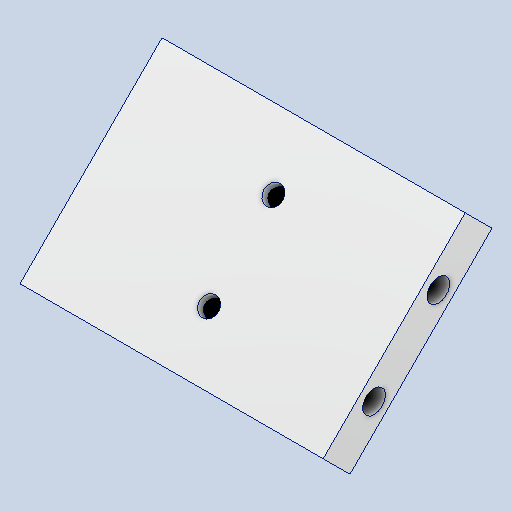
# Autodesk Inventor part: belt_liner_v1_Plate_7
Saved by Autodesk Inventor 2025.2 (Build 292293000, 293)
## iProperties
Created: 2024-12-08
Part Number: belt_liner_v1_Plate_7
Material: アルミニウム 6061
Document SubType Name: Modeling
Designer: haruy
Density: 2.7 g/cm^3
Appearance: アルミニウム - フラット
Author: haruy
Autodesk Inventor part; units mm, degrees
ref_plane "YZ Plane" through (0, 0, 0) normal (1, 0, 0) x (0, 1, 0)
ref_plane "XZ Plane" through (0, 0, 0) normal (0, 1, 0) x (-1, 0, 0)
ref_plane "XY Plane" through (0, 0, 0) normal (0, 0, 1) x (1, 0, 0)
derived "belt_liner_v1_Sketch_Base.ipt"
ref_plane "作業平面3" through (0, 300, 0) normal (0, 1, 0) x (-1, 0, 0)
sketch "スケッチ1" plane through (300, 0, 0) normal (1, 0, 0) x (0, 1, 0)
  circle A0 centre (0, 0) radius 23.875 projected
  circle A1 centre (323.2892, -323.2892) radius 23.875 projected
  line L0 (0, 0) -> (0, -985.832) projected
  line L1 (14.1421, 50.3106) -> (24.7487, 60.9172) projected
  line L2 (24.7487, 60.9172) -> (406.5864, -320.9204) projected
  line L3 (406.5864, -320.9204) -> (395.9798, -331.527) projected
  line L4 (395.9798, -331.527) -> (14.1421, 50.3106) projected
  line L5 (0, 0) -> (323.2892, -323.2892) projected
  line L6 (-50.3106, -14.1421) -> (-60.9172, -24.7487) projected
  line L7 (-60.9172, -24.7487) -> (289.1006, -374.7666) projected
  line L8 (289.1006, -374.7666) -> (299.7072, -364.16) projected
  line L9 (299.7072, -364.16) -> (-50.3106, -14.1421) projected
  line L10 (22.5524, 63.1136) -> (22.5524, 63.1136) projected
  line L11 (14.1421, 50.3106) -> (71.3109, -6.8581) projected
  line L12 (71.3109, -6.8581) -> (67.7754, -10.3937) projected
  line L13 (67.7754, -10.3937) -> (10.6066, 46.7751) projected
  line L14 (10.6066, 46.7751) -> (14.1421, 50.3106) projected
  line L15 (395.9798, -331.527) -> (376.5344, -312.0816) projected
  line L16 (376.5344, -312.0816) -> (372.9988, -315.6171) construction
  line L17 (372.9988, -315.6171) -> (392.4443, -335.0625) construction
  line L18 (392.4443, -335.0625) -> (395.9798, -331.527) projected
  line L19 (0, -985.832) -> (0, 0) projected
  circle A2 centre (0, 0) radius 12.5 projected
  circle A3 centre (21.2132, -21.2132) radius 23.5 construction
  circle A4 centre (0, 0) radius 15 projected
  circle A5 centre (21.2132, -21.2132) radius 15 projected
  line L20 (0, 0) -> (0, 0) projected
  circle A6 centre (-21.2132, 21.2132) radius 15 construction
  circle A7 centre (-21.2132, 21.2132) radius 12.25 construction
  circle A8 centre (0, 0) radius 25.575 construction
  line L21 (0, 0) -> (0, 0) projected
  line L22 (0, 0) -> (0, 0) projected
  circle A9 centre (52.7132, -21.2132) radius 1.5 projected
  circle A10 centre (21.2132, -21.2132) radius 31.5 construction
  line L23 (21.2132, -21.2132) -> (49.9041, 7.4777) projected
  circle A11 centre (21.2132, 10.2868) radius 1.5 projected
  circle A12 centre (-10.2868, -21.2132) radius 1.5 projected
  circle A13 centre (21.2132, -52.7132) radius 1.5 projected
  circle A14 centre (21.2132, -52.7132) radius 3 construction
  circle A15 centre (52.7132, -21.2132) radius 3 construction
  circle A16 centre (21.2132, -52.7132) radius 3 construction
  circle A17 centre (-10.2868, -21.2132) radius 3 construction
  circle A18 centre (21.2132, 10.2868) radius 3 construction
  line L24 (23.3345, 12.4081) -> (54.8345, -19.0919) construction
  line L25 (54.8345, -23.3345) -> (23.3345, -54.8345) construction
  line L26 (19.0919, -54.8345) -> (-12.4081, -23.3345) construction
  line L27 (-50.3106, -14.1421) -> (-46.7751, -10.6066) projected
  line L28 (-46.7751, -10.6066) -> (10.3937, -67.7754) projected
  line L29 (10.3937, -67.7754) -> (6.8581, -71.3109) projected
  line L30 (6.8581, -71.3109) -> (-50.3106, -14.1421) projected
  line L31 (-15.7223, 32.1636) -> (22.5579, 12.9685) construction
  line L32 (-32.1636, 15.7223) -> (-12.9685, -22.5579) construction
  line L33 (84.8528, 0.8132) -> (406.5864, -320.9204) projected
  line L34 (406.5864, -320.9204) -> (410.4755, -317.0313) projected
  line L35 (410.4755, -317.0313) -> (88.7419, 4.7023) projected
  line L36 (88.7419, 4.7023) -> (84.8528, 0.8132) projected
  circle A19 centre (323.2892, -323.2892) radius 5 projected
  line L37 (299.7072, -364.16) -> (280.9689, -345.4217) projected
  line L38 (280.9689, -345.4217) -> (284.5044, -341.8861) projected
  line L39 (284.5044, -341.8861) -> (303.2427, -360.6245) projected
  line L40 (303.2427, -360.6245) -> (299.7072, -364.16) projected
  circle A20 centre (319.7537, -319.7537) radius 5.1 projected
  line L41 (323.2892, -323.2892) -> (417.2615, -417.2615) projected
  circle A21 centre (337.4314, -337.4314) radius 5.1 projected
  line L42 (323.3599, -316.1474) -> (341.0376, -333.8251) projected
  line L43 (316.1474, -323.3599) -> (333.8251, -341.0376) projected
  circle A22 centre (323.2892, -323.2892) radius 22.175 projected
  circle A23 centre (323.2892, -323.2892) radius 33.875 projected
  line L44 (374.5443, -310.0916) -> (356.8667, -327.7692) projected
  line L45 (356.8667, -327.7692) -> (363.9377, -334.8403) projected
  line L46 (363.9377, -334.8403) -> (381.6154, -317.1626) projected
  line L47 (381.6154, -317.1626) -> (374.5443, -310.0916) projected
  circle A24 centre (319.7537, -319.7537) radius 10.1 projected
  circle A25 centre (337.4314, -337.4314) radius 10.1 projected
  line L48 (326.8955, -312.6119) -> (344.5731, -330.2896) projected
  line L49 (312.6119, -326.8955) -> (330.2896, -344.5731) projected
  line L50 (326.8955, -312.6119) -> (318.3599, -304.0764) projected
  line L51 (312.6119, -312.6119) -> (319.7537, -305.4701) projected
  line L52 (319.7537, -305.4701) -> (376.5344, -312.0816) construction
  line L53 (392.4443, -335.0625) -> (303.2427, -360.6245) construction
  line L54 (344.5731, -330.2896) -> (351.3689, -337.0853) projected
  line L55 (351.3689, -337.0853) -> (351.6442, -337.3606) projected
  line L56 (71.3109, -6.8581) -> (67.7754, -10.3937) projected
  line L57 (67.7754, -10.3937) -> (90.8632, -33.4815) projected
  line L58 (90.8632, -33.4815) -> (94.3988, -29.946) projected
  line L59 (94.3988, -29.946) -> (71.3109, -6.8581) projected
  line L60 (244.0828, -334.7487) -> (-45.9172, -334.7487) projected
  line L61 (-45.9172, -334.7487) -> (-45.9172, -349.7487) projected
  line L62 (-45.9172, -349.7487) -> (244.0828, -349.7487) projected
  line L63 (244.0828, -349.7487) -> (244.0828, -334.7487) projected
  line L64 (-60.9172, -24.7487) -> (-60.9172, -604.2835) projected
  line L65 (-45.9172, -334.7487) -> (-60.9172, -334.7487) projected
  line L66 (-60.9172, -334.7487) -> (-60.9172, -349.7487) projected
  line L67 (-60.9172, -349.7487) -> (-45.9172, -349.7487) projected
  line L68 (-45.9172, -349.7487) -> (-45.9172, -334.7487) projected
  line L69 (-60.9172, -334.7487) -> (-45.9172, -334.7487) projected
  line L70 (-45.9172, -334.7487) -> (-45.9172, -44.7487) projected
  line L71 (-45.9172, -44.7487) -> (-60.9172, -44.7487) projected
  line L72 (-60.9172, -44.7487) -> (-60.9172, -334.7487) projected
  line L73 (330.2896, -344.5731) -> (344.5731, -330.2896) projected
  line L74 (344.5731, -330.2896) -> (351.6442, -337.3606) projected
  line L75 (351.6442, -337.3606) -> (337.3606, -351.6442) projected
  line L76 (337.3606, -351.6442) -> (330.2896, -344.5731) projected
  line L77 (406.5864, -320.9204) -> (395.9798, -331.527) projected
  line L78 (395.9798, -331.527) -> (410.1219, -345.6691) projected
  line L79 (410.1219, -345.6691) -> (420.7285, -335.0625) projected
  line L80 (420.7285, -335.0625) -> (406.5864, -320.9204) projected
  line L81 (-12.1904, 2.7649) -> (-50.3106, -35.3553) projected
  line L82 (-12.1904, 2.7649) -> (35.3553, 50.3106) projected
  line L83 (6.8581, -71.3109) -> (-3.7485, -81.9175) projected
  line L84 (-22.0264, -35.3553) -> (-36.1685, -49.4975) construction
  line L85 (-0.8132, -56.5685) -> (-14.9553, -70.7107) projected
  circle A26 centre (-30.8652, -30.052) radius 1.5 construction
  circle A27 centre (-13.1875, -47.7297) radius 1.5 construction
  circle A28 centre (2.7224, -63.6396) radius 1.5 construction
  line L86 (49.4975, 36.1685) -> (35.3553, 22.0264) projected
  line L87 (70.7107, 14.9553) -> (56.5685, 0.8132) projected
  circle A29 centre (40.6586, 20.2586) radius 1.5 projected
  circle A30 centre (58.3363, 2.5809) radius 1.5 projected
  circle A31 centre (63.6396, -2.7224) radius 1.5 construction
  line L88 (289.4542, -346.8359) -> (285.9186, -350.3714) projected
  line L89 (297.9394, -355.3212) -> (294.4039, -358.8567) projected
  circle A32 centre (287.6864, -348.6036) radius 1.5 projected
  circle A33 centre (296.1717, -357.0889) radius 1.5 projected
  line L90 (381.4841, -317.0313) -> (377.9486, -320.5669) construction
  line L91 (389.9694, -325.5166) -> (386.4339, -329.0521) construction
  circle A34 centre (379.7163, -318.7991) radius 1.5 construction
  circle A35 centre (388.2016, -327.2844) radius 1.5 construction
  line L92 (284.5044, -341.8861) -> (312.4678, -312.7589) projected
  line L93 (312.6119, -326.8955) -> (305.4745, -320.0433) projected
  circle A36 centre (333.8958, -323.1478) radius 1.25 projected
  circle A37 centre (323.1478, -333.8958) radius 1.25 projected
  line L94 (-45.9172, -64.7487) -> (-60.9172, -64.7487) projected
  line L95 (-10.3106, -54.1421) -> (-20.9172, -64.7487) projected
  line L96 (-20.9172, -64.7487) -> (-45.9172, -64.7487) projected
  line L97 (224.0828, -334.7487) -> (224.0828, -349.7487) projected
  line L98 (244.0828, -349.7487) -> (264.0828, -349.7487) projected
  line L99 (264.0828, -349.7487) -> (274.6894, -339.1421) projected
  line L100 (244.0828, -334.7487) -> (249.0828, -334.7487) projected
  line L101 (249.0828, -334.7487) -> (259.6894, -324.1421) projected
  line L102 (-45.9172, -44.7487) -> (-40.9172, -44.7487) projected
  line L103 (-40.9172, -44.7487) -> (-30.3106, -34.1421) projected
  line L104 (-45.9172, -329.7487) -> (-60.9172, -329.7487) projected
  line L105 (-25.9172, -334.7487) -> (-25.9172, -349.7487) projected
  line L106 (-24.8548, -32.5269) -> (-38.9969, -46.669) projected
  circle A38 centre (0, 0) radius 45 projected
  circle A39 centre (56.9618, -18.8508) radius 22 projected
  circle A40 centre (56.9618, -18.8508) radius 15 projected
  circle A41 centre (79.5495, -33.4815) radius 3 projected
  circle A42 centre (39.0845, -39.0845) radius 3 projected
  circle A43 centre (39.0845, -39.0845) radius 4 projected
  circle A44 centre (18.8508, -56.9618) radius 22 projected
  circle A45 centre (18.8508, -56.9618) radius 15 projected
  circle A46 centre (33.4815, -79.5495) radius 3 projected
  circle A47 centre (39.0845, -39.0845) radius 3 projected
  line L107 (10.3937, -67.7754) -> (6.8581, -71.3109) projected
  line L108 (6.8581, -71.3109) -> (29.946, -94.3988) projected
  line L109 (29.946, -94.3988) -> (33.4815, -90.8632) projected
  line L110 (33.4815, -90.8632) -> (10.3937, -67.7754) projected
  line L111 (90.8632, -33.4815) -> (33.4815, -90.8632) projected
  circle A48 centre (76.014, -15.0967) radius 1.5 projected
  circle A49 centre (-20.2586, -40.6586) radius 1.5 projected
  circle A50 centre (-2.5809, -58.3363) radius 1.5 projected
  circle A51 centre (15.0967, -76.014) radius 1.5 projected
  circle A52 centre (323.2892, -323.2892) radius 6 projected
  circle A53 centre (0, 0) radius 25.575 construction
  circle A54 centre (0, 0) radius 25.525 projected
  circle A55 centre (323.2892, -323.2892) radius 25.525 projected
  line L112 (341.3381, -305.2403) -> (18.0489, 18.0489) projected
  circle A56 centre (309.7835, -309.7835) radius 4 projected
  circle A57 centre (309.7835, -309.7835) radius 1.25 projected
  circle A58 centre (323.2892, -323.2892) radius 18.525 projected
  circle A59 centre (332.5523, -314.1675) radius 4 projected
  line L113 (316.2182, -330.5017) -> (323.3599, -323.3599) projected
  circle A60 centre (332.5523, -314.1675) radius 1.25 projected
  line L114 (319.7537, -305.4701) -> (324.6327, -300.5911) projected
  line L115 (324.6327, -300.5911) -> (356.5232, -332.4816) projected
  line L116 (351.6442, -337.3606) -> (356.5232, -332.4816) projected
  line L117 (324.6327, -300.5911) -> (308.513, -305.9906) projected
  line L118 (300.5911, -324.6327) -> (332.4816, -356.5232) projected
  line L119 (300.5911, -324.6327) -> (305.9906, -308.513) projected
  line L120 (337.3606, -351.6442) -> (332.4816, -356.5232) projected
  circle A61 centre (314.1675, -332.5523) radius 4 projected
  circle A62 centre (314.1675, -332.5523) radius 1.25 projected
  line L121 (88.7419, 4.7023) -> (131.1683, -37.7241) projected
  line L122 (131.1683, -37.7241) -> (134.3503, -34.5422) projected
  line L123 (134.3503, -34.5422) -> (91.9239, 7.8842) projected
  line L124 (91.9239, 7.8842) -> (88.7419, 4.7023) projected
  circle A63 centre (258.094, 18.4908) radius 120 projected
  line L125 (134.3503, -34.5422) -> (77.7817, 22.0264) projected
  line L126 (77.7817, 22.0264) -> (81.3173, 25.5619) projected
  line L127 (81.3173, 25.5619) -> (137.8858, -31.0066) projected
  line L128 (137.8858, -31.0066) -> (134.3503, -34.5422) projected
  line L129 (76.7211, -47.6236) -> (112.0764, -12.2683) construction
  line L130 (112.0764, -12.2683) -> (119.1475, -19.3394) projected
  line L131 (119.1475, -19.3394) -> (83.7922, -54.6947) construction
  line L132 (83.7922, -54.6947) -> (76.7211, -47.6236) construction
  line L133 (258.094, 18.4908) -> (258.094, 138.4908) projected
  line L134 (258.094, 18.4908) -> (173.2412, 103.3437) projected
  line L135 (258.094, 18.4908) -> (138.094, 18.4908) projected
  line L136 (77.7817, 22.0264) -> (94.3988, -29.946) construction
  circle A64 centre (258.094, 18.4908) radius 130 projected
  line L137 (81.3173, 25.5619) -> (267.9719, 212.2165) projected
  line L138 (258.094, 138.4908) -> (138.094, 18.4908) projected
  line L139 (258.094, 138.4908) -> (258.094, 148.4908) projected
  line L140 (258.094, 18.4908) -> (166.1701, -73.433) projected
  line L141 (173.2412, -66.362) -> (166.1701, -73.433) projected
  line L142 (166.1701, -73.433) -> (180.3122, -87.5752) projected
  line L143 (180.3122, -87.5752) -> (187.3833, -80.5041) projected
  line L144 (187.3833, -80.5041) -> (173.2412, -66.362) projected
  line L145 (180.3122, -87.5752) -> (101.4698, -37.017) construction
  line L146 (410.1219, -345.6691) -> (388.9087, -324.4559) projected
  line L147 (388.9087, -324.4559) -> (385.3732, -327.9915) projected
  line L148 (385.3732, -327.9915) -> (406.5864, -349.2047) projected
  line L149 (406.5864, -349.2047) -> (410.1219, -345.6691) projected
  circle A65 centre (394.212, -333.2948) radius 1.25 projected
  circle A66 centre (401.2831, -340.3658) radius 1.25 projected
  line L150 (120.2082, -20.4) -> (127.2792, -27.4711) projected
  line L151 (127.2792, -27.4711) -> (91.9239, -62.8264) projected
  line L152 (91.9239, -62.8264) -> (84.8528, -55.7554) projected
  line L153 (84.8528, -55.7554) -> (120.2082, -20.4) projected
  line L154 (104.2983, -36.3099) -> (111.3693, -43.381) projected
  line L155 (104.2983, -36.3099) -> (77.7817, 22.0264) projected
  line L156 (111.3693, -43.381) -> (180.3122, -87.5752) projected
  line L157 (90.8632, -33.4815) -> (94.3988, -29.946) projected
  line L158 (94.3988, -29.946) -> (102.5305, -38.0777) projected
  line L159 (102.5305, -38.0777) -> (98.9949, -41.6132) projected
  line L160 (98.9949, -41.6132) -> (90.8632, -33.4815) projected
  line L161 (406.5864, -349.2047) -> (303.2427, -360.6245) projected
  line L162 (319.7537, -305.4701) -> (388.9087, -324.4559) projected
  line L163 (399.5153, -342.1336) -> (413.6575, -327.9915) projected
  circle A67 centre (86.6206, 16.7231) radius 1.25 projected
  circle A68 centre (93.6916, 9.652) radius 1.25 projected
  circle A69 centre (114.9049, -11.5612) radius 1.25 projected
  circle A70 centre (246.5565, 142.9573) radius 1.5 projected
  line L164 (258.094, 138.4908) -> (138.094, 18.4908) projected
  line L165 (138.094, 18.4908) -> (145.165, 11.4198) projected
  line L166 (145.165, 11.4198) -> (265.165, 131.4198) projected
  line L167 (265.165, 131.4198) -> (258.094, 138.4908) projected
  line L168 (258.094, 138.4908) -> (248.452, 148.1328) projected
  line L169 (235.8662, 146.5765) -> (251.0229, 131.4198) projected
  circle A71 centre (258.094, 18.4908) radius 125 projected
  line L170 (138.094, 18.4908) -> (128.452, 28.1328) projected
  circle A72 centre (133.6276, 30.0283) radius 1.5 projected
  line L171 (130.0084, 40.7186) -> (145.165, 25.5619) projected
  point P0 (318.3599, -304.0764)
  point P1 (-53.4172, -334.7487)
  point P2 (287.6864, -348.6036)
  point P3 (-53.4172, -49.7487)
  point P4 (-53.4172, -59.7487)
  point P5 (-29.451, -45.6084)
  point P6 (-22.3799, -52.6795)
  point P7 (239.0828, -342.2487)
  point P8 (229.0828, -342.2487)
  point P9 (224.0828, -342.2487)
  point P10 (266.1196, -341.179)
  point P11 (259.0486, -334.108)
  point P12 (-45.9172, -342.2487)
  point P13 (-53.4172, -344.7487)
  point P14 (-53.4172, -334.7487)
  point P15 (-40.9172, -342.2487)
  point P16 (-30.9172, -342.2487)
  point P17 (39.0845, -39.0845)
  point P18 (69.5431, -8.6259)
  point P19 (394.212, -333.2948)
  constraints: 1 horizontal alignment, 9 other
extrude "押し出し3" add sketch "スケッチ1" against normal blind 40 contours L39 L88 A32 L9 L38 | L39 L89 A33 L9 L88 A32 | L39 L40 L9 L89 A33
sketch "スケッチ8" plane through (260, 303.2427, -360.6245) normal (0, 0.7071068, 0.7071068) x (1, 0, 0)
  line L0 (40, 0) -> (0, 0) projected
  line L1 (0, -26.5) -> (0, 0) projected
  point P0 (-260, -469.425)
  point P1 (20, -19.5)
  point P2 (20, -7.5)
  dimension "d63" = 7.5
  dimension "d64" = 12
  dimension "d65" = 20
  dimension "d66" = 20
  measures "d63" distance from line of point (20, -7.5) L0
  measures "d64" distance of point (20, -19.5) point (20, -7.5)
  measures "d65" distance from line of point (20, -7.5) L1
  measures "d66" distance from line of point (20, -19.5) L1
hole "穴5" at (280, 289.4542, -346.8359) at (280, 297.9394, -355.3212) direction (0, -0.7071068, -0.7071068) diameter 2.5 depth 5 tip angle 118
sketch "スケッチ2" plane through (0, 0, 300) normal (0, 0, 1) x (1, 0, 0)
  circle A0 centre (0, 0) radius 120 projected
  circle A1 centre (-88.3883, -88.3883) radius 5 projected
  circle A2 centre (88.3883, -88.3883) radius 5 projected
  line L0 (0, 0) -> (0, -186.3039) projected
  line L1 (-10, 30) -> (10, 30) projected
  line L2 (10, 30) -> (10, -30) projected
  line L3 (10, -30) -> (-10, -30) projected
  line L4 (-10, -30) -> (-10, 30) projected
  line L5 (12, 2.5) -> (17, 2.5) projected
  line L6 (17, 2.5) -> (17, -2.5) projected
  line L7 (17, -2.5) -> (12, -2.5) projected
  line L8 (12, -2.5) -> (12, 2.5) projected
  circle A3 centre (-88.3883, -88.3883) radius 15 projected
  circle A4 centre (88.3883, -88.3883) radius 15 projected
  circle A5 centre (-7.5, -20) radius 1.5 projected
  circle A6 centre (-7.5, -10) radius 1.5 projected
  circle A7 centre (7.5, -10) radius 1.5 projected
  circle A8 centre (7.5, -20) radius 1.5 projected
  line L9 (0, 0) -> (10, 0) projected
  circle A9 centre (-7.5, 10) radius 1.5 projected
  circle A10 centre (-7.5, 20) radius 1.5 projected
  circle A11 centre (7.5, 10) radius 1.5 projected
  circle A12 centre (7.5, 20) radius 1.5 projected
  line L10 (12, 2.5) -> (17, 2.5) projected
  line L11 (17, 2.5) -> (17, 12.5) projected
  line L12 (17, 12.5) -> (12, 12.5) projected
  line L13 (12, 12.5) -> (12, 2.5) projected
  line L14 (12, -2.5) -> (17, -2.5) projected
  line L15 (17, -2.5) -> (17, -12.5) projected
  line L16 (17, -12.5) -> (12, -12.5) projected
  line L17 (12, -12.5) -> (12, -2.5) projected
  circle A13 centre (14.5, 7.5) radius 1.5 projected
  circle A14 centre (14.5, -7.5) radius 1.5 projected
  circle A15 centre (-14.5, 7.5) radius 1.5 projected
  circle A16 centre (-14.5, -7.5) radius 1.5 projected
  line L18 (-103.0529, -91.5429) -> (-117.3163, -25.2364) projected
  line L19 (-91.5429, -103.0529) -> (-25.2364, -117.3163) projected
  line L20 (91.5429, -103.0529) -> (25.2364, -117.3163) projected
  line L21 (103.0529, -91.5429) -> (117.3163, -25.2364) projected
  circle A17 centre (0, 0) radius 130 projected
  circle A18 centre (0, 0) radius 140 projected
  line L22 (0, 0) -> (137.8731, -24.3107) projected
  line L23 (0, 0) -> (47.8828, -131.557) projected
  line L24 (0, 0) -> (121.2436, -70) projected
  circle A19 centre (46.1727, -126.8585) radius 1.5 projected
  circle A20 centre (116.9134, -67.5) radius 1.5 projected
  circle A21 centre (-46.1727, -126.8585) radius 1.5 projected
  circle A22 centre (-116.9134, -67.5) radius 1.5 projected
  line L25 (0, 0) -> (-137.8731, -24.3107) projected
  circle A23 centre (0, 0) radius 50 projected
  line L26 (-137.8731, -24.3107) -> (-25.6957, 42.8921) projected
  line L27 (137.8731, -24.3107) -> (25.6957, 42.8921) projected
  line L28 (-119.9818, -48) -> (119.9818, -48) projected
  line L29 (119.9818, -48) -> (119.9818, -58) projected
  line L30 (119.9818, -58) -> (-119.9818, -58) projected
  line L31 (-119.9818, -58) -> (-119.9818, -48) construction
  line L32 (-119.9818, -58) -> (-109.9818, -58) projected
  line L33 (-109.9818, -58) -> (-109.9818, -48) projected
  line L34 (-109.9818, -48) -> (-119.9818, -48) projected
  line L35 (-119.9818, -48) -> (-119.9818, -58) construction
  line L36 (119.9818, -58) -> (109.9818, -58) projected
  line L37 (109.9818, -58) -> (109.9818, -48) projected
  line L38 (109.9818, -48) -> (119.9818, -48) projected
  line L39 (119.9818, -48) -> (119.9818, -58) projected
  line L40 (-119.9818, -48) -> (-35.0872, 35.6214) projected
  line L41 (119.9818, -48) -> (35.0872, 35.6214) projected
  circle A24 centre (-70, -53) radius 1.5 projected
  circle A25 centre (-30, -53) radius 1.5 projected
  line L42 (-119.9818, -58) -> (-120, -58) projected
  line L43 (-120, -58) -> (-120, -48) projected
  line L44 (-120, -48) -> (-119.9818, -48) projected
  line L45 (-119.9818, -48) -> (-119.9818, -58) construction
  circle A26 centre (70, -53) radius 1.5 projected
  circle A27 centre (30, -53) radius 1.5 projected
  line L46 (120, -48) -> (119.9818, -48) projected
  line L47 (120, -58) -> (120, -48) projected
  line L48 (119.9818, -58) -> (120, -58) projected
sketch "スケッチ3" plane through (0, 300, 0) normal (0, 1, 0) x (-1, 0, 0)
  circle A0 centre (0, 0) radius 120 projected
  line L0 (-120, 256.5601) -> (-120, -448.0203) projected
  line L1 (-120, 57.9583) -> (-110, 57.9583) projected
  line L2 (-110, 57.9583) -> (-110, 47.9583) projected
  line L3 (-110, 47.9583) -> (-120, 47.9583) projected
  line L4 (-120, 47.9583) -> (-120, 57.9583) projected
  line L5 (-110, 57.9583) -> (120, 57.9583) projected
  line L6 (120, 57.9583) -> (120, 47.9583) projected
  line L7 (120, 47.9583) -> (-110, 47.9583) projected
  line L8 (-110, 47.9583) -> (-110, 57.9583) projected
  constraints: 1 other
ref_plane "作業平面1" through (300, 0, 0) normal (1, 0, 0) x (0, 1, 0)
ref_plane "作業平面2" through (0, 0, 300) normal (0, 0, 1) x (1, 0, 0)
equation "\"d66\" = d65"
